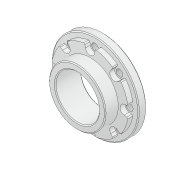
# Autodesk Inventor part: 16_029_X430_FREE_HORN_R1
Saved by Autodesk Inventor 2021 (Build 250183000, 183)
## iProperties
Created: 2020-07-25
Part Number: 16_029_X430_FREE_HORN_R1
Material: Aluminum 6061
Document SubType Name: Modeling
Designer: y6tada
Density: 2.7 g/cm^3
Appearance: Aluminum - Flat
Author: y6tada
Autodesk Inventor part; units mm, degrees
ref_plane "YZ Plane" through (0, 0, 0) normal (1, 0, 0) x (0, 1, 0)
ref_plane "XZ Plane" through (0, 0, 0) normal (0, 1, 0) x (-1, 0, 0)
ref_plane "XY Plane" through (0, 0, 0) normal (0, 0, 1) x (1, 0, 0)
sketch "Sketch1" plane through (0, 0, 0) normal (0, 0, 1) x (1, 0, 0)
  point P0 (0, 0)
sketch "Sketch2" plane through (0, 0, 0) normal (0, 0, 1) x (1, 0, 0)
  circle A0 centre (0, 0) radius 5
  circle A1 centre (0, 0) radius 10
  circle A2 centre (0, 0) radius 8 construction
  line L0 (0, 0) -> (8, 0) construction
  dimension "d2" = 16
  dimension "d0" = 10
  dimension "d1" = 20
  constraints: 4 coincident, 2 centre point, 2 end point, 1 horizontal, 1 horizontal alignment, 2 other
  measures "d0" diameter of A0
  measures "d1" diameter of A1
extrude "Extrusion1" add sketch "Sketch2" along normal blind 6
sketch "Sketch3" plane through (0, 0, 6) normal (0, 0, 1) x (1, 0, 0)
  circle A0 centre (0, 0) radius 6.5
  circle A1 centre (0, 0) radius 10 projected
  dimension "d5" = 13
  constraints: 1 centre point, 1 coincident
  measures "d5" diameter of A0
extrude "Extrusion2" cut sketch "Sketch3" against normal blind 3
sketch "Sketch4" plane through (0, 0, 3) normal (0, 0, 1) x (1, 0, 0)
  circle A0 centre (0, 0) radius 8.8
  circle A1 centre (0, 0) radius 10 projected
  dimension "d8" = 17.6
  constraints: 1 centre point, 1 coincident
  measures "d8" diameter of A0
extrude "Extrusion3" cut sketch "Sketch4" against normal blind 1.15
sketch "Sketch5" plane through (0, 0, 3) normal (0, 0, 1) x (1, 0, 0)
  line L0 (0, 0) -> (8, 0) construction
  circle A0 centre (0, 0) radius 8 construction
  line L1 (8, 0) -> (10, 0) construction
  line L2 (7.8487, -1.0896) -> (9.8109, -1.3619)
  line L3 (9.8109, 1.3619) -> (7.8487, 1.0896)
  arc A1 (7.8487, 1.0896) -> (7.8487, -1.0896) centre (8, 0) ccw
  arc A2 (9.8109, -1.3619) -> (9.8109, 1.3619) centre (10, 0) ccw
  line L4 (7.8487, 1.0896) -> (0, 0) construction
  circle A3 centre (0, 0) radius 10 construction
  point P0 (9, 0)
  dimension "d11" = 16
  dimension "d12" = 1.1
  constraints: 12 end point, 4 point on circle, 4 tangent, 2 centre point, 2 coincident, 2 horizontal, 2 horizontal alignment, 1 collinear, 1 midpoint, 3 other
  measures "d12" radius of A1
extrude "Extrusion4" cut sketch "Sketch5" against normal up to surface (1.15 mm away)
fillet "Fillet1" radius 0.25 2 edges at (8.7164, -1.21, 2.425) (8.7164, 1.21, 2.425)
hole "Hole1" at (8, 0, 3) direction (0, 0, -1) diameter 1.567 end through all thread size "M2x0.4" class "6H" standard "ANSI Metric M Profile"
pattern_circular "Circular Pattern1" count 8 over 360 about axis through (0, 0, -10) along (0, 0, 1) of "Extrusion4", "Fillet1", "Hole1"
chamfer "Chamfer1" distance 0.2 angle 45 5 edges at (-5, 0, 6) (-5, 0, 0) (-6.5, 0, 6) (-10, 0, 0) (-10, 0, 1.85)
body "Solid1"
